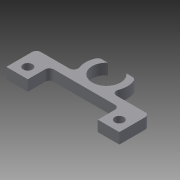
# Autodesk Inventor part: BearingSupport
Saved by Autodesk Inventor 2014 SP1 (Build 180222100, 222)
## iProperties
Created: 2017-05-20
Part Number: BearingSupport
Material: Generic
Document SubType Name: Modeling
Designer: danielsikar
Density: 1 g/cm^3
Appearance: Default
Author: danielsikar
Autodesk Inventor part; units mm, degrees
ref_plane "YZ Plane" through (0, 0, 0) normal (1, 0, 0) x (0, 1, 0)
ref_plane "XZ Plane" through (0, 0, 0) normal (0, 1, 0) x (-1, 0, 0)
ref_plane "Work Plane5" through (-24.85, -3.5, 5) normal (0, 0, 1) x (1, 0, 0)
sketch "Sketch16" plane through (-24.85, -3.5, 5) normal (0, 0, 1) x (1, 0, 0)
  circle A0 centre (0, 0) radius 6.5 construction
  arc A1 (-8.312, 5) -> (8.312, 5) centre (0, 0) ccw
  line L0 (9.7, 0) -> (-9.7, 0) construction
  line L1 (8.312, 5) -> (-8.312, 5)
  arc A2 (-4.3933, 4.9254) -> (4.3933, 4.9254) centre (0, 0) ccw
  arc A3 (-4.3081, 5) -> (4.3081, 5) centre (0, 0) ccw
  point P0 (24.85, 3.5)
  point P1 (4.4598, 5)
  point P2 (-4.4598, 5)
  dimension "d45" = 5
  constraints: 8 point on circle, 4 end point, 4 point on line, 3 centre point, 1 coincident, 1 concentric, 1 horizontal, 1 parallel
  measures "d45" distance between parallel lines of L1 L0
extrude "Extrusion16" add sketch "Sketch16" against normal blind 5 contours L1 A3 A2 A1
sketch "Sketch17" plane through (-24.85, -3.5, 5) normal (0, 0, 1) x (1, 0, 0)
  circle A0 centre (-21.25, -15.25) radius 2.15 projected
  circle A1 centre (21.25, -15.25) radius 2.15 projected
  arc A2 (-24.25, -6.25) -> (-26.25, -8.25) centre (-24.25, -8.25) ccw projected
  line L0 (-23.35, -6.25) -> (-24.25, -6.25) projected
  arc A3 (-23.35, -6.25) -> (-21.35, -4.25) centre (-23.35, -4.25) ccw projected
  line L1 (-21.35, -0.6245) -> (-21.35, -4.25) projected
  arc A4 (-21.35, -0.6245) -> (-21.35, 0.6245) centre (-19.45, 0) ccw projected
  line L2 (-21.35, 4.25) -> (-21.35, 0.6245) projected
  arc A5 (-19.35, 6.25) -> (-21.35, 4.25) centre (-19.35, 4.25) ccw projected
  line L3 (-19.35, 6.25) -> (-16.95, 6.25) projected
  line L4 (-16.95, 6.25) -> (-16.95, -6.25) projected
  line L5 (-16.95, -6.25) -> (6.65, -6.25) projected
  line L6 (6.65, -6.25) -> (6.65, 6.25) projected
  line L7 (6.65, 6.25) -> (9.05, 6.25) projected
  arc A6 (11.05, 4.25) -> (9.05, 6.25) centre (9.05, 4.25) ccw projected
  line L8 (11.05, 4.25) -> (11.05, 0.6245) projected
  arc A7 (11.05, 0.6245) -> (11.05, -0.6245) centre (9.15, 0) ccw projected
  line L9 (11.05, -0.6245) -> (11.05, -4.25) projected
  arc A8 (11.05, -4.25) -> (13.05, -6.25) centre (13.05, -4.25) ccw projected
  line L10 (13.05, -6.25) -> (24.25, -6.25) projected
  arc A9 (26.25, -8.25) -> (24.25, -6.25) centre (24.25, -8.25) ccw projected
  line L11 (26.25, -8.25) -> (26.25, -20.25) projected
  arc A10 (16.25, -12.25) -> (14.25, -10.25) centre (14.25, -12.25) ccw projected
  line L12 (14.25, -10.25) -> (-14.25, -10.25) projected
  arc A11 (-14.25, -10.25) -> (-16.25, -12.25) centre (-14.25, -12.25) ccw projected
  line L13 (-26.25, -20.25) -> (-26.25, -8.25) projected
  line L14 (-16.25, -12.25) -> (-16.25, -20.25) projected
  line L15 (-26.25, -20.25) -> (-16.25, -20.25) projected
  line L16 (16.25, -20.25) -> (26.25, -20.25) projected
  line L17 (16.25, -12.25) -> (16.25, -20.25) projected
  point P0 (24.85, 3.5)
extrude "Extrusion17" add sketch "Sketch17" against normal blind 5
sketch "Sketch18" plane through (-24.85, -3.5, 0) normal (0, 0, -1) x (-1, 0, 0)
  line L0 (16.95, -6.25) -> (7.4181, -6.25) projected
  line L1 (14.25, -6.25) -> (26.25, -6.25)
  line L2 (26.25, -6.25) -> (26.25, 6.25)
  line L3 (26.25, 6.25) -> (14.25, 6.25)
  line L4 (14.25, 6.25) -> (14.25, -6.25)
  point P0 (-24.85, 3.5)
  constraints: 8 end point, 2 parallel, 1 horizontal, 1 perpendicular, 1 point on line
extrude "Extrusion18" cut sketch "Sketch18" against normal blind 5
sketch "Sketch19" plane through (-24.85, -3.5, 0) normal (0, 0, -1) x (-1, 0, 0)
  line L0 (-4.4598, 5) -> (-15.1519, 5)
  line L1 (-15.1519, 5) -> (-15.1519, 7.7901)
  line L2 (-15.1519, 7.7901) -> (-4.4598, 7.7901)
  line L3 (-4.4598, 7.7901) -> (-4.4598, 5)
  point P0 (-24.85, 3.5)
  constraints: 8 end point, 2 parallel, 1 horizontal, 1 perpendicular
extrude "Extrusion19" cut sketch "Sketch19" against normal blind 5
sketch "Sketch20" plane through (-24.85, -3.5, 0) normal (0, 0, -1) x (-1, 0, 0)
  line L0 (-4.3081, 5) -> (-10.904, 5) projected
  arc A0 (-13.05, -6.25) -> (-11.05, -4.25) centre (-13.05, -4.25) ccw projected
  line L1 (-14.25, -10.25) -> (14.25, -10.25) projected
  line L2 (24.25, -6.25) -> (7.4181, -6.25) projected
  line L3 (8.312, 5) -> (4.3081, 5) projected
  line L4 (-6.65, -0.817) -> (-6.65, 0.817) projected
  arc A1 (-4.4598, 5) -> (-6.65, 0.817) centre (0, 0) ccw projected
  line L5 (-7.14, 5) -> (-12.1327, 5)
  line L6 (-13.05, -6.25) -> (-7.4181, -6.25)
  arc A2 (-8.1939, -10.25) -> (11.5386, -6.25) centre (0, 0) ccw
  arc A3 (-12.1327, 5) -> (-11.5386, -6.25) centre (0, 0) ccw
  arc A4 (7.4181, -6.25) -> (8.312, 5) centre (0, 0) ccw
  arc A5 (-8.312, 5) -> (-7.4181, -6.25) centre (0, 0) ccw
  point P0 (4.4598, 5)
  point P1 (-24.85, 3.5)
  constraints: 9 point on circle, 6 end point, 5 point on line, 4 centre point, 1 coincident, 1 parallel, 1 perpendicular
extrude "Extrusion20" cut sketch "Sketch20" against normal blind 5 contours A5 L6 A3 L5 L0
sketch "Sketch21" plane through (-24.85, -3.5, 0) normal (0, 0, -1) x (-1, 0, 0)
  line L0 (-13.05, -6.25) -> (-24.25, -6.25) projected
  line L1 (-15.1128, -6.25) -> (-9.6695, -6.25)
  line L2 (-9.6695, -6.25) -> (-9.6695, -4.6771)
  line L3 (-9.6695, -4.6771) -> (-15.1128, -4.6771)
  line L4 (-15.1128, -4.6771) -> (-15.1128, -6.25)
  point P0 (-24.85, 3.5)
  constraints: 8 end point, 2 parallel, 1 horizontal, 1 perpendicular, 1 point on line
extrude "Extrusion21" cut sketch "Sketch21" against normal blind 5
fillet "Fillet2" radius 2 4 edges at (-17.4319, -9.75, 2.5) (-33.162, 1.5, 2.5) (-16.538, 1.5, 2.5) (-32.2681, -9.75, 2.5)
sketch "Sketch22" plane through (-24.85, -3.5, 0) normal (0, 0, -1) x (-1, 0, 0)
  line L0 (7.0915, 5) -> (4.3081, 5) projected
  line L1 (2.1207, -6.25) -> (-2.1207, -6.25) projected
  line L2 (-6.65, -0.817) -> (-6.65, 0.817) projected
  line L3 (-2.414, -6.25) -> (2.414, -6.25)
  arc A0 (-4.3081, 5) -> (-2.1207, -6.25) centre (0, 0) ccw construction
  arc A1 (2.1207, -6.25) -> (4.3081, 5) centre (0, 0) ccw construction
  arc A2 (-2.1207, -6.25) -> (2.1207, -6.25) centre (0, 0) ccw
  point P0 (4.4598, 5)
  point P1 (-24.85, 3.5)
  constraints: 4 end point, 3 point on line, 2 point on circle, 1 centre point, 1 coincident, 1 collinear, 1 concentric
extrude "Extrusion23" cut sketch "Sketch22" against normal blind 5
body "Solid3"
